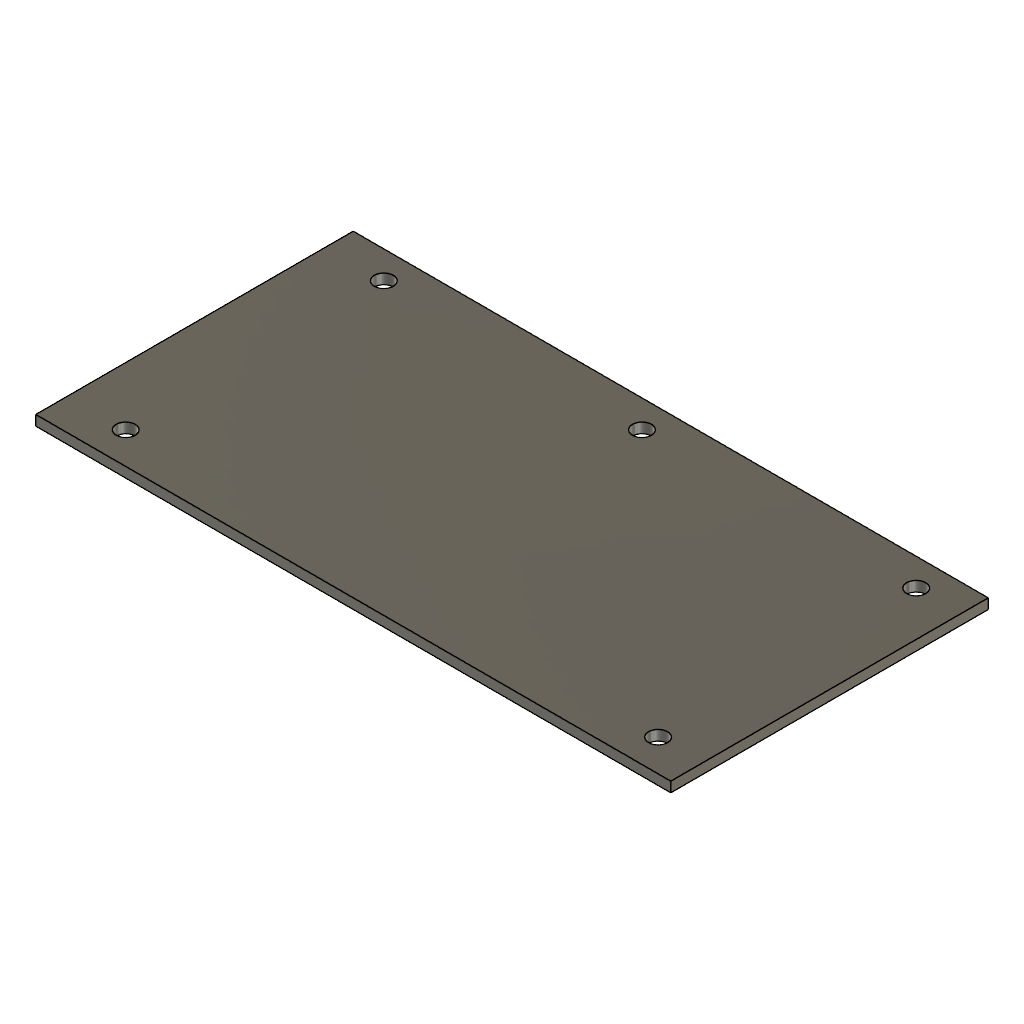
Platine (Autodesk Fusion 360 design; units mm, degrees)
Autodesk Fusion 360 part; units mm, degrees
sketch "Skizze1" plane through (0, 0, 0) normal (0, 0, 1) x (1, 0, 0)
  line L0 (-100, 50) -> (0, 50)
  line L1 (0, 50) -> (0, 0)
  line L2 (0, 0) -> (-100, 0)
  line L3 (-100, 0) -> (-100, 50)
  line L4 (-100, 45.64) -> (0, 45.64) construction
  line L5 (-100, 5) -> (0, 5) construction
  line L6 (-7, 50) -> (-7, 0) construction
  line L7 (-90.82, 50) -> (-90.82, 0) construction
  line L8 (-50.18, 50) -> (-50.18, 0) construction
  circle A0 centre (-90.82, 5) radius 1.5
  circle A1 centre (-90.82, 45.64) radius 1.5
  circle A2 centre (-7, 45.64) radius 1.5
  circle A3 centre (-7, 5) radius 1.5
  circle A4 centre (-50.18, 45.64) radius 1.5
  line L9 (-12.08, 50) -> (-12.08, 0) construction
  line L10 (-88.28, 50) -> (-88.28, 0) construction
  line L11 (-12.08, 20.24) -> (-88.28, 20.24) construction
  line L12 (-12.08, 32.94) -> (-88.28, 32.94) construction
  line L13 (-90.82, 12.62) -> (-7, 12.62) construction
  line L14 (-90.82, 38.02) -> (-7, 38.02) construction
  line L15 (-60.34, 38.02) -> (-60.34, 12.62) construction
  line L16 (-70.5, 45.64) -> (-70.5, 5) construction
  line L17 (-83.2, 45.64) -> (-83.2, 5) construction
  line L18 (-70.5, 35.48) -> (-83.2, 35.48) construction
  line L19 (-70.5, 15.16) -> (-83.2, 15.16) construction
  point P0 (-12.08, 20.24)
  point P1 (-12.08, 32.94)
  point P2 (-88.28, 32.94)
  point P3 (-88.28, 20.24)
  point P4 (-7, 38.02)
  point P5 (-7, 12.62)
  point P6 (-60.34, 38.02)
  point P7 (-60.34, 12.62)
  point P8 (-70.5, 35.48)
  point P9 (-70.5, 15.16)
  point P10 (-83.2, 15.16)
  point P11 (-83.2, 35.48)
  dimension "d1" = 100
  dimension "d2" = 50
  dimension "d3" = 5
  dimension "d4" = 7
  dimension "d5" = 83.82
  dimension "d6" = 40.64
  dimension "d7" = 3
  dimension "d9" = 5.08
  dimension "d10" = 2.54
  dimension "d11" = 12.7
  dimension "d14" = 25.4
  dimension "d15" = 5.08
  dimension "d16" = 12.7
  dimension "d17" = 53.34
  dimension "d19" = 10.16
  dimension "d20" = 12.7
  dimension "d21" = 2.54
  dimension "d22" = 2.54
  dimension "d29" = 40.64
  constraint horizontal L0
  constraint vertical L1
  constraint horizontal L2
  constraint vertical L3
  constraint coincident L1.end L2.start
  constraint coincident L3 L4.start
  constraint perpendicular L3 L4
  constraint coincident L3 L5.start
  constraint coincident L1 L5.end
  constraint perpendicular L1 L5
  constraint coincident L0 L6.start
  constraint coincident L2 L6.end
  constraint perpendicular L2 L6
  constraint coincident L0 L7.start
  constraint coincident L2 L7.end
  constraint perpendicular L2 L7
  constraint coincident L0 L8.start
  constraint coincident L2 L8.end
  constraint coincident L7 A0.centre
  constraint coincident L5 A0.centre
  constraint coincident L7 A1.centre
  constraint coincident L4 A1.centre
  constraint coincident L6 A2.centre
  constraint coincident L4 A2.centre
  constraint coincident L6 A3.centre
  constraint coincident L5 A3.centre
  constraint equal A2 A3
  constraint equal A1 A2
  constraint equal A0 A1
  constraint vertical L8
  constraint coincident L8 A4.centre
  constraint coincident L4 A4.centre
  constraint equal A2 A4
  constraint coincident L0 L9.start
  constraint coincident L2 L9.end
  constraint perpendicular L2 L9
  constraint coincident L0 L10.start
  constraint coincident L2 L10.end
  constraint perpendicular L2 L10
  constraint coincident L9 P0
  constraint coincident L9 P1
  constraint coincident P0 L11.start
  constraint coincident L10 P3
  constraint perpendicular L10 L11
  constraint coincident P1 L12.start
  constraint coincident L10 P2
  constraint perpendicular L10 L12
  constraint coincident P2 L12.end
  constraint coincident P3 L11.end
  constraint coincident L7 L13.start
  constraint coincident L6 P5
  constraint perpendicular L6 L13
  constraint coincident L7 L14.start
  constraint perpendicular L9 L14
  constraint coincident L6 P4
  constraint coincident P4 L14.end
  constraint coincident P5 L13.end
  constraint coincident L14 P6
  constraint coincident P6 L15.start
  constraint coincident L13 P7
  constraint perpendicular L13 L15
  constraint coincident P7 L15.end
  constraint coincident L4 L16.start
  constraint coincident L5 L16.end
  constraint perpendicular L5 L16
  constraint coincident L4 L17.start
  constraint coincident L5 L17.end
  constraint perpendicular L5 L17
  constraint coincident L16 P8
  constraint coincident L17 P11
  constraint perpendicular L17 L18
  constraint coincident L16 P9
  constraint coincident L17 P10
  constraint perpendicular L17 L19
  constraint coincident P8 L18.start
  constraint coincident P9 L19.start
  constraint coincident P10 L19.end
  constraint coincident P11 L18.end
  measures "d1" distance of L1.end L2.end
  measures "d2" distance of L0.end L1.end
  measures "d3" distance of L2 L5
  measures "d4" distance of L1 L6
  measures "d5" distance of L6 L7
  measures "d6" distance of L4 L5
  measures "d7" diameter of A3
  measures "d9" distance of L6 L9
  measures "d10" distance of L7 L10
  measures "d11" distance of P0 P1
  measures "d14" distance of L13 L14
  measures "d15" distance of L12 L14
  measures "d16" distance of L4 L12
  measures "d17" distance of P4 P6
  measures "d19" distance of P6 L16
  measures "d20" distance of L16 L17
  measures "d21" distance of L14 L18
  measures "d22" distance of L13 L19
  measures "d29" distance of A1.centre A4.centre
extrude "Extrusion1" add sketch "Skizze1" along normal blind 1.6
ref_plane "Arbeitsebene1" through (-50, 25, 12.6) normal (0, 0, 1) x (1, 0, 0)
sketch "Skizze2" plane through (0, 0, 12.6) normal (0, 0, 1) x (1, 0, 0)
  point P0 (-7, 38.02)
  point P1 (-7, 12.62)
  point P2 (-60.34, 38.02)
  point P3 (-60.34, 12.62)
  point P4 (-88.28, 32.94)
  point P5 (-88.28, 20.24)
ref_plane "Arbeitsebene2" through (-50, 25, -11) normal (0, 0, 1) x (1, 0, 0)
sketch "Skizze3" plane through (0, 0, -11) normal (0, 0, 1) x (1, 0, 0)
  point P0 (-83.2, 15.16)
  point P1 (-70.5, 15.16)
  point P2 (-70.5, 35.48)
  point P3 (-83.2, 35.48)
  point P4 (-12.08, 20.24)
  point P5 (-12.08, 32.94)
equation "d5 = 33 * 2.54 mm"
equation "d9 = ( 2 * 2.54 ) * 1 mm"
equation "d11 = ( 5 * 2.54 ) * 1 mm"
equation "d14 = ( 10 * 2.54 ) * 1 mm"
equation "d15 = 2 * 2.54 mm"
equation "d16 = ( 5 * 2.54 ) * 1 mm"
equation "d17 = ( 21 * 2.54 ) * 1 mm"
equation "d19 = ( 4 * 2.54 ) * 1 mm"
equation "d20 = ( 5 * 2.54 ) * 1 mm"
equation "d29 = ( 16 * 2.54 ) * 1 mm"
